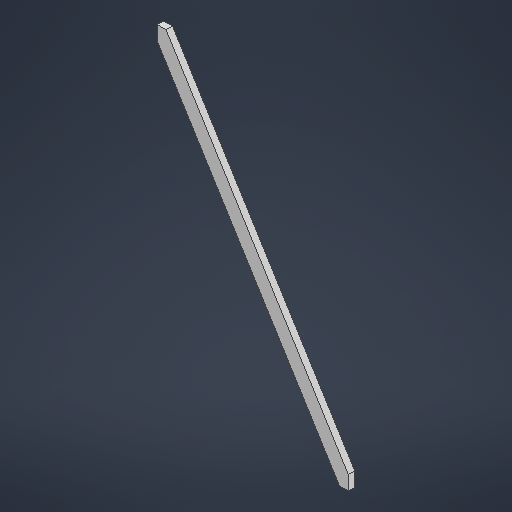
# Autodesk Inventor part: S_2x4x84.708
Saved by Autodesk Inventor 2026 (Build 300175000, 175)
## iProperties
Created: 2025-09-05
Part Number: S_2x4x84.708
Material: Generic
Document SubType Name: Modeling
Designer: trott
Density: 1 g/cm^3
Appearance: Default
Author: trott
Autodesk Inventor part; units mm, degrees
ref_plane "YZ Plane" through (0, 0, 0) normal (1, 0, 0) x (0, 1, 0)
ref_plane "XZ Plane" through (0, 0, 0) normal (0, 1, 0) x (-1, 0, 0)
ref_plane "XY Plane" through (0, 0, 0) normal (0, 0, 1) x (1, 0, 0)
sketch "Sketch1" plane through (0, 0, 0) normal (0, 0, 1) x (1, 0, 0)
  line L0 (-1152.525, 0) -> (1152.525, 0)
  line L1 (-19.05, 0) -> (19.05, 0)
  line L2 (-19.05, 0) -> (-19.05, 1828.8)
  line L3 (19.05, 0) -> (19.05, 1828.8)
  line L4 (19.05, 1828.8) -> (-19.05, 1828.8)
  line L5 (1152.525, 0) -> (1152.525, 1828.8)
  line L6 (1152.525, 1828.8) -> (19.05, 1828.8)
  line L7 (-1152.525, 0) -> (-1152.525, 1828.8)
  line L8 (-1152.525, 1828.8) -> (-19.05, 1828.8)
  line L9 (-1152.525, 1828.8) -> (-19.05, 0)
  line L10 (19.05, 0) -> (1152.525, 1828.8)
  line L11 (-56.8317, -23.4168) -> (18.7317, 23.4168)
  line L12 (-1190.3067, 1805.3832) -> (-1114.7433, 1852.2168)
  line L13 (-1190.3067, 1805.3832) -> (-56.8317, -23.4168)
  line L14 (18.7317, 23.4168) -> (-1114.7433, 1852.2168)
  line L15 (0, 1828.8) -> (0, 0)
  point P0 (-19.05, 84.3755)
  point P1 (-1100.2298, 1828.8)
  point P2 (-1152.525, 1744.4245)
  point P3 (-71.3452, 0)
  dimension "d0" = 2305.05
  dimension "d1" = 38.1
  dimension "d2" = 1828.8
  dimension "d3" = 1828.8
  dimension "d4" = 1828.8
  dimension "d5" = 1828.8
  dimension "d6" = 88.9
  dimension "d7" = 88.9
  constraints: 32 end point, 5 midpoint, 4 perpendicular, 3 point on line, 1 horizontal, 1 vertical
  measures "d0" distance of L0.start L0.end
  measures "d1" distance of L1.start L1.end
  measures "d2" distance of L1.start L2.end
  measures "d3" distance of L1.end L3.end
  measures "d4" distance of L0.end L5.end
  measures "d5" distance of L0.start L7.end
  measures "d6" distance of L11.start L11.end
  measures "d7" distance of L12.start L12.end
extrude "Extrusion1" add sketch "Sketch1" along normal blind 38.1 contours L9 L8 L14 L2 | L0 L13 L7 L9
body "Solid1"
